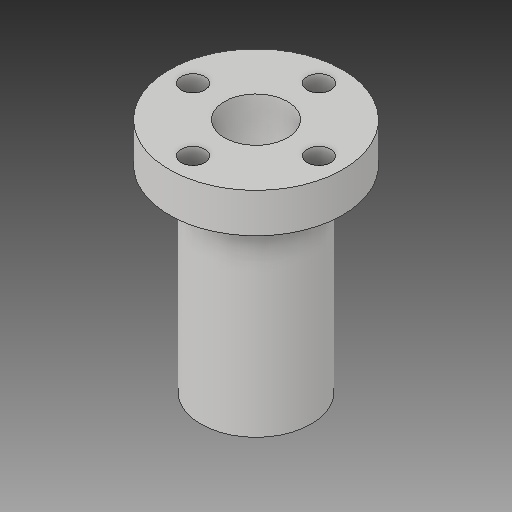
# Autodesk Inventor part: standinNut
Saved by Autodesk Inventor 2019 (Build 230136000, 136)
## iProperties
Created: 2019-05-07
Part Number: standinNut
Material: Generic
Document SubType Name: Modeling
Designer: Alex Jones
Density: 1 g/cm^3
Appearance: Default
Mass: 4.09978 g
Surface Area: 29.9651 cm^2
Volume: 4.09978 cm^3
Author: Alex Jones
Autodesk Inventor part; units mm, degrees
ref_plane "YZ Plane" through (0, 0, 0) normal (1, 0, 0) x (0, 1, 0)
ref_plane "XZ Plane" through (0, 0, 0) normal (0, 1, 0) x (-1, 0, 0)
sketch "Sketch1" plane through (0, 0, 0) normal (1, 0, 0) x (0, 1, 0)
  line L0 (0, 0) -> (-84.9068, 0)
  line L1 (0, -4) -> (-84.9068, -4)
  line L2 (0, -4) -> (0, -11)
  line L3 (0, -11) -> (-5, -11)
  line L4 (-5, -11) -> (-5, -7)
  line L5 (-5, -7) -> (-30, -7)
  line L6 (-30, -7) -> (-30, -4)
  dimension "d1" = 4
  dimension "d2" = 11
  dimension "d3" = 5
  dimension "d4" = 4
  dimension "d5" = 25
  constraints: 14 end point, 3 horizontal, 2 vertical, 1 parallel, 1 perpendicular, 1 point on line
  measures "d1" distance between parallel lines of L0 L1
  measures "d2" distance of L0.start L2.end
  measures "d3" distance of L2.end L3.end
  measures "d4" distance of L3.end L4.end
  measures "d5" distance of L4.end L5.end
revolve "Revolution1" add sketch "Sketch1" angle 360 about axis through (0, 0, 0) along (0, -1, 0)
sketch "Sketch2" plane through (0, -5, 0) normal (0, -1, 0) x (1, 0, 0)
  line L0 (0, 0) -> (8, 0)
  circle A0 centre (8, 0) radius 1.5
  circle A1 centre (0, 8) radius 1.5
  circle A2 centre (-8, 0) radius 1.5
  circle A3 centre (0, -8) radius 1.5
  dimension "d7" = 8
  dimension "d8" = 3
  dimension "d11" = 360
  constraints: 4 centre point, 2 end point, 1 coincident, 1 horizontal, 9 other
  measures "d7" distance of L0.start L0.end
  measures "d8" diameter of A0
extrude "Extrusion1" cut sketch "Sketch2" against normal blind 25.4
ref_plane "Work Plane1" through (-8, -5, 0) normal (0, 0, -1) x (0, 1, 0)
body "Solid1"
